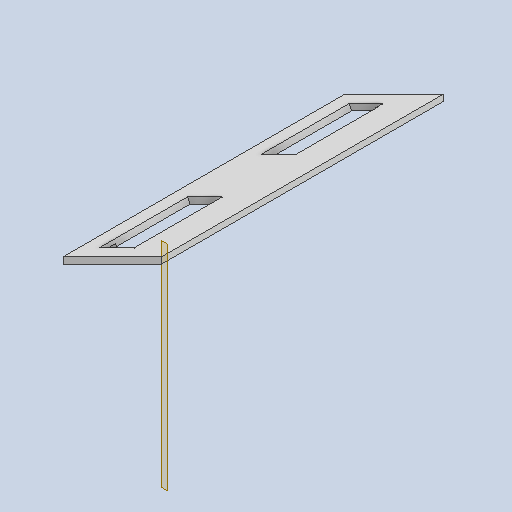
# Autodesk Inventor part: pług_v2
Saved by Autodesk Inventor 2023 (Build 270158000, 158)
## iProperties
Created: 2022-10-17
Part Number: pług_v2
Material: Generic
Document SubType Name: Modeling
Designer: komputer
Density: 1 g/cm^3
Appearance: Default
Author: komputer
Autodesk Inventor part; units mm, degrees
ref_plane "YZ Plane" through (0, 0, 0) normal (1, 0, 0) x (0, 1, 0)
ref_plane "XZ Plane" through (0, 0, 0) normal (0, 1, 0) x (-1, 0, 0)
ref_plane "XY Plane" through (0, 0, 0) normal (0, 0, 1) x (1, 0, 0)
ref_plane "Work Plane1" through (0, 0, 0) normal (0, 0, 1) x (1, 0, 0)
sketch "Sketch1" plane through (0, 0, 0) normal (0, 0, 1) x (1, 0, 0)
  line L0 (-15.4497, 44.5138) -> (-27.4258, 43.3684) projected
  arc A0 (-37, -19.9971) -> (-36.2161, -20.9735) centre (-36, -19.9971) ccw projected
  line L1 (-36.2161, -20.9735) -> (-23.4006, -23.8092) projected
  arc A1 (-23.4006, -23.8092) -> (-22.2674, -22.4343) centre (-23.1845, -22.8329) ccw projected
  arc A2 (-15.124, -1.2705) -> (-22.2674, -22.4343) centre (-7, -15.8) ccw projected
  arc A3 (-2, 0) -> (-15.124, -1.2705) centre (-7, -16.7705) ccw projected
  line L2 (-2, 0) -> (-2, 61.9933) projected
  arc A4 (-2, 61.9933) -> (-4.8944, 63.7822) centre (-4, 61.9933) ccw projected
  line L3 (-4.8944, 63.7822) -> (-17.5444, 57.4573) projected
  arc A5 (-17.5444, 57.4573) -> (-17.9916, 56.1156) centre (-17.0971, 56.5628) ccw projected
  line L4 (-17.9916, 56.1156) -> (-16.2204, 52.5733) projected
  line L5 (-16.2204, 52.5733) -> (-15.4497, 44.5138) projected
  line L6 (-5.7149, 25.9193) -> (-9.7149, 25.9193) projected
  line L7 (-9.7149, 25.9193) -> (-9.7149, 32.3193) projected
  line L8 (-9.7149, 32.3193) -> (-5.7149, 32.3193) projected
  line L9 (-5.7149, 32.3193) -> (-5.7149, 25.9193) projected
  circle A6 centre (-14.1745, 5.2514) radius 1.25 projected
  circle A7 centre (-12.3575, 40.5948) radius 1.25 projected
  line L10 (0, 0) -> (0, 69) projected
  line L11 (0, 69) -> (-2, 69) projected
  line L12 (-2, 0) -> (-2, 69) projected
  line L13 (0, 0) -> (-2, 0) projected
  line L14 (-2, 65.2294) -> (-36.7798, 47.8397)
  line L15 (-2, 65.2294) -> (-2.8944, 67.0182)
  line L16 (-37, 24.9335) -> (-37.5, 24.9335)
  line L17 (-37.5, 24.9335) -> (-37.5, 47.4795)
  line L18 (-37.5, 47.4795) -> (-37, 47.4795)
  line L19 (-37, 47.4795) -> (-37, 24.9335)
  line L20 (-37, 47.4795) -> (-37.5, 47.4795)
  line L21 (-37.5, 47.4795) -> (-37.5, 51.8841)
  line L22 (-37.5, 51.8841) -> (-37, 51.8841)
  line L23 (-37, 51.8841) -> (-37, 47.4795)
  line L24 (-36.7798, 47.8397) -> (-39.9927, 46.2332)
  line L25 (-37, 47.7295) -> (-37.8944, 49.5184)
  line L26 (-37.8944, 49.5184) -> (-2.8944, 67.0182)
  line L27 (-37, 47.7295) -> (-37, 49.9656)
  line L28 (-2, 65.2294) -> (-2, 67.4654)
  line L29 (-2.8944, 67.0182) -> (-2, 67.4654)
  line L30 (-16.3638, 38.7424) -> (-30.4647, 38.7424) projected
  arc A8 (-26.2111, 2.9303) -> (-25.4939, 4.574) centre (-29.8942, 5.5158) ccw projected
  line L31 (-37, 47.0432) -> (-37, -19.9971) projected
  line L32 (-27.4258, 43.3684) -> (-28.2236, 51.7105) projected
  line L33 (-28.2236, 51.7105) -> (-37, 47.0432) projected
  arc A9 (-30.8142, -5.934) -> (-31.4006, -7.3529) centre (-21.8926, -10.4512) ccw projected
  arc A10 (-33.794, -6.9728) -> (-31.4006, -7.3529) centre (-32.5671, -6.9728) ccw projected
  line L34 (-33.794, -6.9728) -> (-30.8638, 38.3682) projected
  arc A11 (-30.4647, 38.7424) -> (-30.8638, 38.3682) centre (-30.4647, 38.3424) ccw projected
  arc A12 (-15.9789, 38.2336) -> (-16.3638, 38.7424) centre (-16.3638, 38.3424) ccw projected
  line L35 (-15.9789, 38.2336) -> (-25.4939, 4.574) projected
  arc A13 (-26.2111, 2.9303) -> (-26.948, 1.702) centre (-18.0264, -2.8152) ccw projected
  line L36 (-26.948, 1.702) -> (-30.8142, -5.934) projected
  point P0 (-24.3837, 38.7424)
  dimension "d0" = 2
  dimension "d1" = 0.5
  dimension "d2" = 2
  constraints: 32 end point, 7 point on line, 4 parallel, 4 perpendicular, 2 collinear, 2 horizontal
  measures "d0" distance of L14.start L15.end
  measures "d1" distance of L17.end L18.end
  measures "d2" distance of L25.start L25.end
extrude "Extrusion1" add sketch "Sketch1" against normal blind 100 contours L14 L24 L23 L26 L15 L3 | L15 L29 L12
sketch "Sketch2" plane through (-2, 67.4654, 0) normal (-0.44721, 0.894429, 0) x (0.894429, 0.44721, 0)
  line L0 (-21.6579, 7.5484) -> (-21.306, 16.8472) projected
  line L1 (-20.8996, 27.5881) -> (-20.5477, 36.8868) projected
  line L2 (-20.5477, 36.8868) -> (-23.0666, 36.8868) projected
  line L3 (-29.9704, 36.8868) -> (-32.4893, 36.8868) projected
  line L4 (-33.5995, 7.5484) -> (-32.4893, 36.8868) projected
  line L5 (-21.8658, 16.8472) -> (-22.195, 8.1452) projected
  line L6 (-21.306, 16.8472) -> (-21.8658, 16.8472) projected
  line L7 (-21.6579, 7.5484) -> (-21.306, 16.8472) projected
  line L8 (-21.6579, 7.5484) -> (-24.1768, 7.5484) projected
  line L9 (-24.1768, 7.5484) -> (-24.316, 3.8687) projected
  ellipse E0 centre (-27.7679, 3.8687) end of major axis (-28.8048, 0.317) minor radius 3.433 (-31.2198, 3.8687) -> (-24.316, 3.8687) ccw projected
  line L10 (-31.0806, 7.5484) -> (-31.2198, 3.8687) projected
  line L11 (-31.0806, 7.5484) -> (-33.5995, 7.5484) projected
  line L12 (-33.5995, 7.5484) -> (-32.4893, 36.8868) projected
  line L13 (-29.9704, 36.8868) -> (-32.4893, 36.8868) projected
  line L14 (-29.9704, 36.8868) -> (-29.8312, 40.5666) projected
  ellipse E1 centre (-26.3793, 40.5666) end of major axis (-27.4161, 37.0148) minor radius 3.433 (-22.9274, 40.5666) -> (-29.8312, 40.5666) ccw projected
  line L15 (-23.0666, 36.8868) -> (-22.9274, 40.5666) projected
  line L16 (-20.5477, 36.8868) -> (-23.0666, 36.8868) projected
  line L17 (-20.8996, 27.5881) -> (-20.5477, 36.8868) projected
  line L18 (-21.4593, 27.5881) -> (-20.8996, 27.5881) projected
  line L19 (-21.13, 36.2901) -> (-21.4593, 27.5881) projected
  line L20 (-31.9522, 36.2901) -> (-21.13, 36.2901) projected
  line L21 (-31.9522, 36.2901) -> (-33.0172, 8.1452) projected
  line L22 (-33.0172, 8.1452) -> (-22.195, 8.1452) projected
  ellipse E2 centre (-27.7698, 3.819) end of major axis (-28.2182, 2.2831) minor radius 1.4845 projected
  ellipse E3 centre (-26.3774, 40.6163) end of major axis (-26.8258, 39.0804) minor radius 1.4845 projected
  line L23 (-27.4544, 6.3673) -> (-26.3442, 35.7057) projected
  line L24 (-19.711, 6.3673) -> (-27.4544, 6.3673) projected
  line L25 (-18.6008, 35.7057) -> (-19.711, 6.3673) projected
  line L26 (-26.3442, 35.7057) -> (-18.6008, 35.7057) projected
  line L27 (-26.7698, 14.5969) -> (-27.052, 7.138) projected
  line L28 (-19.7727, 14.5969) -> (-26.7698, 14.5969) projected
  line L29 (-19.7727, 14.5969) -> (-20.055, 7.138) projected
  line L30 (-20.055, 7.138) -> (-27.052, 7.138) projected
  line L31 (-19.0031, 34.9349) -> (-26.0002, 34.9349) projected
  line L32 (-19.0031, 34.9349) -> (-19.6166, 18.7242) projected
  line L33 (-19.6166, 18.7242) -> (-26.6136, 18.7242) projected
  line L34 (-26.0002, 34.9349) -> (-26.6136, 18.7242) projected
  line L35 (-26.3442, 64.2943) -> (-27.4544, 93.6327) projected
  line L36 (-18.6008, 64.2943) -> (-26.3442, 64.2943) projected
  line L37 (-19.711, 93.6327) -> (-18.6008, 64.2943) projected
  line L38 (-27.4544, 93.6327) -> (-19.711, 93.6327) projected
  line L39 (-26.2824, 72.524) -> (-26.0002, 65.0651) projected
  line L40 (-19.2854, 72.524) -> (-26.2824, 72.524) projected
  line L41 (-19.2854, 72.524) -> (-19.0031, 65.0651) projected
  line L42 (-19.0031, 65.0651) -> (-26.0002, 65.0651) projected
  line L43 (-20.055, 92.862) -> (-27.052, 92.862) projected
  line L44 (-20.055, 92.862) -> (-19.4416, 76.6513) projected
  line L45 (-19.4416, 76.6513) -> (-26.4386, 76.6513) projected
  line L46 (-27.052, 92.862) -> (-26.4386, 76.6513) projected
  line L47 (-21.4593, 72.4119) -> (-21.13, 63.7099) projected
  line L48 (-20.8996, 72.4119) -> (-21.4593, 72.4119) projected
  line L49 (-20.5477, 63.1132) -> (-20.8996, 72.4119) projected
  line L50 (-20.5477, 63.1132) -> (-23.0666, 63.1132) projected
  line L51 (-23.0666, 63.1132) -> (-22.9274, 59.4334) projected
  ellipse E4 centre (-26.3793, 59.4334) end of major axis (-25.3424, 55.8817) minor radius 3.433 (-29.8312, 59.4334) -> (-22.9274, 59.4334) ccw projected
  line L52 (-29.9704, 63.1132) -> (-29.8312, 59.4334) projected
  line L53 (-29.9704, 63.1132) -> (-32.4893, 63.1132) projected
  line L54 (-32.4893, 63.1132) -> (-33.5995, 92.4516) projected
  line L55 (-31.0806, 92.4516) -> (-33.5995, 92.4516) projected
  line L56 (-31.0806, 92.4516) -> (-31.2198, 96.1313) projected
  ellipse E5 centre (-27.7679, 96.1313) end of major axis (-26.7311, 92.5795) minor radius 3.433 (-24.316, 96.1313) -> (-31.2198, 96.1313) ccw projected
  line L57 (-24.1768, 92.4516) -> (-24.316, 96.1313) projected
  line L58 (-21.6579, 92.4516) -> (-24.1768, 92.4516) projected
  line L59 (-21.306, 83.1528) -> (-21.6579, 92.4516) projected
  line L60 (-21.8658, 83.1528) -> (-21.306, 83.1528) projected
  line L61 (-22.195, 91.8548) -> (-21.8658, 83.1528) projected
  line L62 (-33.0172, 91.8548) -> (-22.195, 91.8548) projected
  line L63 (-33.0172, 91.8548) -> (-31.9522, 63.7099) projected
  line L64 (-31.9522, 63.7099) -> (-21.13, 63.7099) projected
  ellipse E6 centre (-26.3774, 59.3837) end of major axis (-25.929, 57.8478) minor radius 1.4845 projected
  ellipse E7 centre (-27.7698, 96.181) end of major axis (-27.3214, 94.6451) minor radius 1.4845 projected
  line L65 (-18.6008, 35.7057) -> (-27.4544, 35.7057)
  line L66 (-27.4544, 35.7057) -> (-27.4544, 6.3673)
  line L67 (-27.4544, 6.3673) -> (-18.6008, 6.3673)
  line L68 (-18.6008, 6.3673) -> (-18.6008, 35.7057)
  line L69 (-27.4544, 6.3673) -> (-28.4544, 6.3673)
  line L70 (-28.4544, 6.3673) -> (-28.4544, 5.7086)
  line L71 (-28.4544, 5.7086) -> (-27.4544, 5.7086)
  line L72 (-27.4544, 5.7086) -> (-27.4544, 6.3673)
  line L73 (-18.6008, 35.7057) -> (-17.6008, 35.7057)
  line L74 (-17.6008, 35.7057) -> (-17.6008, 36.8868)
  line L75 (-17.6008, 36.8868) -> (-18.6008, 36.8868)
  line L76 (-18.6008, 36.8868) -> (-18.6008, 35.7057)
  line L77 (-17.6008, 36.8868) -> (-28.4544, 36.8868)
  line L78 (-28.4544, 36.8868) -> (-28.4544, 5.7086)
  line L79 (-28.4544, 5.7086) -> (-17.6008, 5.7086)
  line L80 (-17.6008, 5.7086) -> (-17.6008, 36.8868)
  point P0 (-28.3824, 0)
  point P1 (-27.4544, 8.1452)
  point P2 (-27.3871, 8.1452)
  point P3 (-28.4544, 6.3673)
  point P4 (-27.4544, 5.7086)
  point P5 (-17.6008, 35.7057)
  point P6 (-18.6008, 36.8868)
  dimension "d5" = 1
  dimension "d6" = 1
  constraints: 32 end point, 8 parallel, 4 horizontal, 4 perpendicular, 6 other
  measures "d5" distance of L71.end L70.end
  measures "d6" distance of L75.end L74.end
extrude "Extrusion2" cut sketch "Sketch2" against normal blind 3 contours L8 L9 L30 L27 L22 L5 L28 L0 | L0 L28 L29 L30 L9 L8 | L28 L5 L6 L0 | L0 L6 L5 L28 L27 L22 L23 L26 L19 L31 L34 L33 L32 L1 L25 L24 L9 L30 L29 | L5 L22 L27 L28 | L9 L24 L23 L22 L27 L30 | L24 L67 L68 L73 L80 L79 L9 | L9 L79 L72 L24 | L25 L68 L67 | L69 L78 L22 L66 | L72 L71 L70 L69 | L22 L66 L65 L23 | L76 L75 L74 L73 | L26 L1 L77 L76 | L22 L78 L20 L19 L26 L65 L66 | L26 L19 L20 L78 L77 L2 L1 | L1 L31 L19 L26 | L31 L32 L33 L34 L19 L18 L1 | L1 L18 L19 L31
sketch "Sketch3" plane through (-2, 67.4654, 0) normal (-0.44721, 0.894429, 0) x (0.894429, 0.44721, 0)
  line L0 (0, 0) -> (-39.1311, 0) projected
  line L1 (0, 0) -> (0, 100) projected
  line L2 (-39.1311, 100) -> (0, 100) projected
  line L3 (-39.1311, 0) -> (-39.1311, 100) projected
  line L4 (-17.6008, 36.8868) -> (-17.6008, 5.7086) projected
  line L5 (-17.6008, 5.7086) -> (-28.4544, 5.7086) projected
  line L6 (-28.4544, 5.7086) -> (-28.4544, 36.8868) projected
  line L7 (-28.4544, 36.8868) -> (-17.6008, 36.8868) projected
  line L8 (-28.4544, 36.8868) -> (-28.4544, 5.7086) projected
  line L9 (-28.4544, 5.7086) -> (-29.4544, 5.7086)
  line L10 (-29.4544, 5.7086) -> (-29.4544, 36.8868)
  line L11 (-29.4544, 36.8868) -> (-28.4544, 36.8868)
  line L12 (-28.4544, 36.8868) -> (-28.4544, 5.7086)
  line L13 (-28.4544, 36.8868) -> (-29.9544, 36.8868)
  line L14 (-29.9544, 36.8868) -> (-29.9544, 5.7086)
  line L15 (-29.9544, 5.7086) -> (-28.4544, 5.7086)
  line L16 (-28.4544, 5.7086) -> (-28.4544, 36.8868)
  line L17 (-39.1311, 0) -> (-39.1311, 100) projected
  line L18 (-39.1311, 50) -> (0, 50)
  line L19 (0, 0) -> (0, 100) projected
  line L20 (-17.6008, 63.1132) -> (-17.6008, 94.2914)
  line L21 (-17.6008, 94.2914) -> (-28.4544, 94.2914)
  line L22 (-28.4544, 63.1132) -> (-17.6008, 63.1132)
  line L23 (-29.4544, 63.1132) -> (-28.4544, 63.1132)
  line L24 (-28.4544, 63.1132) -> (-29.9544, 63.1132)
  line L25 (-29.9544, 63.1132) -> (-29.9544, 94.2914)
  line L26 (-29.9544, 94.2914) -> (-28.4544, 94.2914)
  point P0 (-28.3824, 0)
  point P1 (-28.4544, 94.2914)
  point P2 (-29.4544, 5.7086)
  dimension "d9" = 1
  dimension "d10" = 1.5
  constraints: 32 end point, 9 symmetric about line, 4 parallel, 2 horizontal, 2 midpoint, 2 perpendicular, 1 point on line
  measures "d9" distance of L10.end L11.end
  measures "d10" distance of L15.end L14.end
extrude "Extrusion3" cut sketch "Sketch3" against normal blind 3 contours L6 L9 L10 L11 | L10 L15 L14 L13 | L22 L23 L24 L25 L26 L21 L20
sketch "Sketch4" plane through (-2, 67.4654, 0) normal (-0.44721, 0.894429, 0) x (0.894429, 0.44721, 0)
  line L0 (-17.6008, 5.7086) -> (-29.9544, 5.7086) projected
  line L1 (-29.9544, 5.7086) -> (-29.9544, 36.8868) projected
  line L2 (-29.9544, 36.8868) -> (-17.6008, 36.8868) projected
  line L3 (-17.6008, 36.8868) -> (-17.6008, 5.7086) projected
  line L4 (0, 0) -> (-39.1311, 0) projected
  line L5 (0, 0) -> (0, 100) projected
  line L6 (-39.1311, 100) -> (0, 100) projected
  line L7 (-39.1311, 0) -> (-39.1311, 100) projected
  line L8 (-29.9544, 94.2914) -> (-17.6008, 94.2914) projected
  line L9 (-17.6008, 94.2914) -> (-17.6008, 63.1132) projected
  line L10 (-17.6008, 63.1132) -> (-29.9544, 63.1132) projected
  line L11 (-29.9544, 63.1132) -> (-29.9544, 94.2914) projected
  line L12 (-17.6008, 5.7086) -> (-29.9544, 5.7086) projected
  line L13 (-29.9544, 5.7086) -> (-30.9544, 5.7086)
  line L14 (-30.9544, 5.7086) -> (-30.9544, 36.8868)
  line L15 (-30.9544, 36.8868) -> (-29.9544, 36.8868)
  line L16 (-29.9544, 36.8868) -> (-29.9544, 5.7086)
  line L17 (-29.9544, 94.2914) -> (-29.9544, 63.1132) projected
  line L18 (-29.9544, 63.1132) -> (-30.9544, 63.1132)
  line L19 (-30.9544, 63.1132) -> (-30.9544, 94.2914)
  line L20 (-30.9544, 94.2914) -> (-29.9544, 94.2914)
  line L21 (-29.9544, 94.2914) -> (-29.9544, 63.1132)
  point P0 (-28.3824, 0)
  point P1 (-29.9544, 94.2914)
  point P2 (-29.9544, 36.8868)
  dimension "d13" = 1
  constraints: 16 end point, 4 parallel, 2 horizontal, 2 perpendicular, 1 point on line
  measures "d13" distance of L14.end L15.end
extrude "Extrusion4" cut sketch "Sketch4" against normal blind 3 contours L13 L14 L15 L1 | L11 L18 L19 L20
sketch "Sketch5" plane through (-2, 67.4654, 0) normal (-0.44721, 0.894429, 0) x (0.894429, 0.44721, 0)
  ellipse E0 centre (-26.3793, 40.5666) end of major axis (-27.4161, 37.0148) minor radius 3.433 (-22.9274, 40.5666) -> (-29.8312, 40.5666) ccw projected
  line L0 (-30.9544, 94.2914) -> (-17.6008, 94.2914) projected
  line L1 (-17.6008, 94.2914) -> (-17.6008, 63.1132) projected
  line L2 (-17.6008, 63.1132) -> (-30.9544, 63.1132) projected
  line L3 (-30.9544, 63.1132) -> (-30.9544, 94.2914) projected
  line L4 (-30.9544, 36.8868) -> (-17.6008, 36.8868) projected
  line L5 (-17.6008, 36.8868) -> (-17.6008, 5.7086) projected
  line L6 (-17.6008, 5.7086) -> (-30.9544, 5.7086) projected
  line L7 (-30.9544, 5.7086) -> (-30.9544, 36.8868) projected
  line L8 (0, 0) -> (-39.1311, 0) projected
  line L9 (0, 0) -> (0, 100) projected
  line L10 (-39.1311, 100) -> (0, 100) projected
  line L11 (-39.1311, 0) -> (-39.1311, 100) projected
  line L12 (-17.6008, 5.7086) -> (-17.1008, 5.7086)
  line L13 (-17.1008, 5.7086) -> (-17.1008, 36.8868)
  line L14 (-17.1008, 36.8868) -> (-17.6008, 36.8868)
  line L15 (-17.6008, 36.8868) -> (-17.6008, 5.7086)
  line L16 (-17.6008, 63.1132) -> (-30.9544, 63.1132) projected
  line L17 (-17.6008, 63.1132) -> (-17.1008, 63.1132)
  line L18 (-17.1008, 63.1132) -> (-17.1008, 91.9206)
  line L19 (-17.1008, 91.9206) -> (-17.6008, 91.9206)
  line L20 (-17.6008, 91.9206) -> (-17.6008, 63.1132)
  point P0 (-28.3824, 0)
  point P1 (-17.6008, 91.9206)
  point P2 (-17.6008, 36.8868)
  dimension "d16" = 0.5
  dimension "d17" = 0.5
  constraints: 16 end point, 4 parallel, 2 horizontal, 2 perpendicular, 1 other
  measures "d16" distance of L14.end L13.end
  measures "d17" distance of L19.end L18.end
extrude "Extrusion5" cut sketch "Sketch5" against normal blind 3 contours L19 L18 L17 L1 | L14 L13 L12 L5
body "Solid1"
